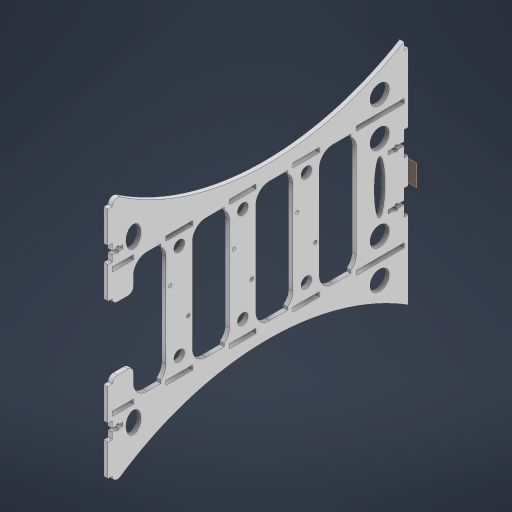
# Autodesk Inventor part: грань тела
Saved by Autodesk Inventor 2023.2 (Build 272271030, 271C)
## iProperties
Created: 2024-11-21
Part Number: грань тела
Material: Типовые
Document SubType Name: Modeling
Designer: DELL
Density: 1 g/cm^3
Appearance: По умолчанию
Author: DELL
Autodesk Inventor part; units mm, degrees
ref_plane "YZ Plane" through (0, 0, 0) normal (1, 0, 0) x (0, 1, 0)
ref_plane "XZ Plane" through (0, 0, 0) normal (0, 1, 0) x (-1, 0, 0)
ref_plane "РабПлоскость1" through (0, 0, -4) normal (0, 0, 1) x (1, 0, 0)
sketch "Эскиз10" plane through (0, 0, 0) normal (1, 0, 0) x (0, 1, 0)
  line L0 (-120, -4) -> (120, -4) construction
  line L1 (120, -4) -> (120, 276) construction
  line L2 (110.389, 276) -> (-110.389, 276)
  line L3 (-120, 276) -> (-120, -4) construction
  line L4 (-110, -4) -> (110, -4)
  arc A0 (-110, -4) -> (-114.5368, 268.208) centre (-321.9309, 128.6096) ccw
  arc A1 (114.5368, 268.208) -> (110, -4) centre (321.9309, 128.6096) ccw
  arc A2 (114.5368, 268.208) -> (110.389, 276) centre (110.389, 271) ccw
  arc A3 (-110.389, 276) -> (-114.5368, 268.208) centre (-110.389, 271) ccw
  point P0 (0, 0)
  point P1 (0, -4)
  dimension "d50" = 240
  dimension "d51" = 280
  dimension "d52" = 220
  dimension "d53" = 250
  dimension "d54" = 250
  dimension "d55" = 5
  constraints: 10 end point, 10 point on circle, 4 centre point, 4 tangent, 2 horizontal, 2 midpoint, 2 parallel, 2 point on line, 1 equal radius, 1 perpendicular
  measures "d50" distance of L3.start L1.end
  measures "d51" distance of L1.end L0.end
  measures "d52" distance of L4.start L4.end
  measures "d53" radius of A0
  measures "d54" radius of A1
  measures "d55" radius of A2
extrude "Выдавливание6" add sketch "Эскиз10" along normal mid plane 4
sketch "Эскиз12" plane through (2, 0, 0) normal (1, 0, 0) x (0, 0, -1)
  line L0 (3.3197, -100.9593) -> (0, -100.9593)
  line L1 (4, 110) -> (4, -110) projected
  line L2 (4, -110) -> (4, 110) projected
  line L3 (4, -35.9593) -> (0, -35.9593)
  line L4 (0, -35.9593) -> (0, -12.5)
  line L5 (0, -12.5) -> (4, -12.5)
  line L6 (4, 12.5) -> (0, 12.5)
  line L7 (0, 12.5) -> (0, 35.5004)
  line L8 (0, 35.5004) -> (4, 35.5004)
  line L9 (0, 100.5004) -> (4, 100.5004)
  line L10 (0, -100.9593) -> (0, -110)
  line L11 (0, -110) -> (4, -110)
  line L12 (0, 100.5004) -> (0, 110)
  line L13 (0, 110) -> (4, 110)
  line L14 (0, -100.9593) -> (0, -50.9593)
  line L15 (0, -50.9593) -> (4, -50.9593)
  line L16 (0, 100.5004) -> (0, 50.5004)
  line L17 (0, 50.5004) -> (4, 50.5004)
  point P0 (0, 0)
  point P1 (4, 12.5)
  point P2 (4, 35.5004)
  point P3 (4, -35.9593)
  point P4 (4, -12.5)
  point P5 (4, -100.9593)
  dimension "d197" = 50
  dimension "d198" = 50
  constraints: 32 end point, 11 perpendicular, 8 point on line, 3 vertical, 1 horizontal, 6 other
  measures "d197" distance of L0.end L14.end
  measures "d198" distance of L9.start L16.end
extrude "Выдавливание7" cut sketch "Эскиз12" against normal blind 4 contours L1 L9 L12 L13 | L1 L6 L7 L8 | L1 L3 L4 L5
sketch "Эскиз13" plane through (2, 0, 0) normal (1, 0, 0) x (0, 0, -1)
  line L0 (-15, -22.6546) -> (-15, -25.8046)
  line L1 (0, -25.7683) -> (0, -22.691)
  line L2 (0, -35.9593) -> (0, -12.5) projected
  line L3 (-6.1608, -27.016) -> (-8.4608, -27.016)
  line L4 (-8.4608, -21.516) -> (-6.1608, -21.516)
  line L5 (-15, -24.2296) -> (0, -24.2296) construction
  line L6 (0, -12.5) -> (0, -35.9593) projected
  line L7 (-8.4608, -27.016) -> (-8.4608, -25.8046)
  line L8 (-8.4608, -22.6546) -> (-8.4608, -21.516)
  line L9 (-15, -25.8046) -> (-8.4608, -25.8046)
  line L10 (-6.1608, -25.7683) -> (0, -25.7683)
  line L11 (-6.1608, -21.516) -> (-6.1608, -22.691)
  line L12 (-6.1608, -25.7683) -> (-6.1608, -27.016)
  line L13 (0, -22.691) -> (-6.1608, -22.691)
  line L14 (-8.4608, -22.6546) -> (-15, -22.6546)
  line L15 (0, 12.5) -> (0, 35.5004) projected
  line L16 (0, 18.7449) -> (0, 30.6124)
  line L17 (0, 22.4252) -> (0, 25.5752)
  line L18 (-15, 25.5752) -> (-15, 22.4252)
  line L19 (-8.65, 21.2502) -> (-6.35, 21.2502)
  line L20 (-6.35, 26.7502) -> (-8.65, 26.7502)
  line L21 (-15, 24.0002) -> (0, 24.0002) construction
  line L22 (-8.65, 26.7502) -> (-8.65, 25.5752)
  line L23 (-8.65, 22.4252) -> (-8.65, 21.2502)
  line L24 (-15, 22.4252) -> (-8.65, 22.4252)
  line L25 (-6.35, 22.4252) -> (0, 22.4252)
  line L26 (-6.35, 21.2502) -> (-6.35, 22.4252)
  line L27 (-6.35, 25.5752) -> (-6.35, 26.7502)
  line L28 (0, 25.5752) -> (-6.35, 25.5752)
  line L29 (-8.65, 25.5752) -> (-15, 25.5752)
  circle A0 centre (-23.1563, -40) radius 9
  line L30 (4, -35.9593) -> (4, -110) projected
  line L31 (4, 35.5004) -> (4, 100.5004) projected
  line L32 (0, 0) -> (-64.5188, 0) construction
  circle A1 centre (-23.1563, 40) radius 9
  point P0 (4, -60.9593)
  point P1 (4, 60.5004)
  dimension "d60" = 15
  dimension "d61" = 3.15
  dimension "d62" = 2.3
  dimension "d63" = 5.5
  dimension "d64" = 6.35
  dimension "d70" = 15
  dimension "d71" = 3.15
  dimension "d72" = 2.3
  dimension "d73" = 5.5
  dimension "d77" = 18
  dimension "d114" = 80
  constraints: 56 end point, 20 parallel, 10 perpendicular, 8 midpoint, 7 horizontal, 2 centre point, 2 point on line, 1 symmetric about line, 1 other
  measures "d60" distance of L1.start L0.end
  measures "d61" distance of L0.end L0.start
  measures "d62" distance of L4.start L4.end
  measures "d63" distance of L3.end L4.start
  measures "d64" distance of point (0, -24.23) L11.end
  measures "d70" distance of L18.start L17.end
  measures "d71" distance of L17.end L17.start
  measures "d72" distance of L20.end L20.start
  measures "d73" distance of L20.start L19.end
  measures "d77" diameter of A0
  measures "d114" distance of A1.centre A0.centre
extrude "Выдавливание8" cut sketch "Эскиз13" against normal blind 4
sketch "Эскиз15" plane through (-2, 0, 0) normal (-1, 0, 0) x (0, 0, 1)
  line L0 (0, 75.3813) -> (0, -75.381) construction
  line L1 (0, 57.0002) -> (0, 61.0002) construction
  line L2 (0, 61.0002) -> (276, 61.0002) construction
  line L3 (276, 61.0002) -> (276, 57.0002) construction
  line L4 (276, 57.0002) -> (0, 57.0002) construction
  line L5 (0, -61.2296) -> (0, -57.2296) construction
  line L6 (0, -57.2296) -> (276, -57.2296) construction
  line L7 (276, -57.2296) -> (276, -61.2296) construction
  line L8 (276, -61.2296) -> (0, -61.2296) construction
  circle A0 centre (23.1563, 40) radius 9 construction
  circle A1 centre (23.1563, -40) radius 9 construction
  line L9 (45.1563, 57.0002) -> (45.1563, -44.2296) construction
  line L10 (118.1563, 57.0002) -> (127.1563, 57.0002)
  line L11 (140.1563, 44.0002) -> (140.1563, -44.2296)
  line L12 (127.1563, -57.2296) -> (118.1563, -57.2296)
  line L13 (105.1563, -44.2296) -> (105.1563, 44.0002)
  line L14 (238.1563, 57.0002) -> (243, 57.0002)
  line L15 (243, -57.2296) -> (238.1563, -57.2296)
  line L16 (225.1563, -44.2296) -> (225.1563, 44.0002)
  line L17 (276, 35.0002) -> (276, 110.389)
  line L18 (178.1563, 57.0002) -> (187.1563, 57.0002)
  line L19 (200.1563, 44.0002) -> (200.1563, -44.2296)
  line L20 (187.1563, -57.2296) -> (178.1563, -57.2296)
  line L21 (165.1563, -44.2296) -> (165.1563, 44.0002)
  line L22 (58.1563, 57.0002) -> (67.1563, 57.0002)
  line L23 (80.1563, 44.0002) -> (80.1563, -44.2296)
  line L24 (67.1563, -57.2296) -> (58.1563, -57.2296)
  line L25 (45.1563, -57.2296) -> (45.1563, 44.0002)
  arc A2 (50.1563, 54.2471) -> (45.1563, 44.0002) centre (58.1563, 44.0002) ccw
  arc A3 (80.1563, 44.0002) -> (67.1563, 57.0002) centre (67.1563, 44.0002) ccw
  arc A4 (45.1563, -44.2296) -> (50.1563, -54.4766) centre (58.1563, -44.2296) ccw
  arc A5 (67.1563, -57.2296) -> (80.1563, -44.2296) centre (67.1563, -44.2296) ccw
  arc A6 (110.1563, 54.2471) -> (105.1563, 44.0002) centre (118.1563, 44.0002) ccw
  arc A7 (140.1563, 44.0002) -> (127.1563, 57.0002) centre (127.1563, 44.0002) ccw
  arc A8 (105.1563, -44.2296) -> (110.1563, -54.4766) centre (118.1563, -44.2296) ccw
  arc A9 (127.1563, -57.2296) -> (140.1563, -44.2296) centre (127.1563, -44.2296) ccw
  arc A10 (170.1563, 54.2471) -> (165.1563, 44.0002) centre (178.1563, 44.0002) ccw
  arc A11 (200.1563, 44.0002) -> (187.1563, 57.0002) centre (187.1563, 44.0002) ccw
  arc A12 (187.1563, -57.2296) -> (200.1563, -44.2296) centre (187.1563, -44.2296) ccw
  arc A13 (165.1563, -44.2296) -> (170.1563, -54.4766) centre (178.1563, -44.2296) ccw
  arc A14 (230.1563, 54.2471) -> (225.1563, 44.0002) centre (238.1563, 44.0002) ccw
  arc A15 (256, 44.0002) -> (243, 57.0002) centre (243, 44.0002) ccw
  arc A16 (243, -57.2296) -> (256, -44.2296) centre (243, -44.2296) ccw
  arc A17 (225.1563, -44.2296) -> (230.1563, -54.4766) centre (238.1563, -44.2296) ccw
  line L26 (271, -29.9962) -> (261, -29.9962)
  line L27 (261, 30.0002) -> (271, 30.0002)
  line L28 (276, -13.2762) -> (255.9998, 30.0002) construction
  line L29 (256.0015, -29.9962) -> (276, 13.2766) construction
  line L30 (276, 41.3488) -> (276, 1056.4994)
  line L31 (276, 110.389) -> (276, -110.389) projected
  arc A18 (271, 30.0002) -> (276, 35.0002) centre (271, 35.0002) ccw
  line L32 (276, -34.9962) -> (276, -49)
  arc A19 (276, -34.9962) -> (271, -29.9962) centre (271, -34.9962) ccw
  line L33 (276, 57.0002) -> (276, -57.2296)
  line L34 (256, 44.0002) -> (256, 35.0002)
  line L35 (256, -34.9962) -> (256, -44.2296)
  arc A20 (256, 35.0002) -> (261, 30.0002) centre (261, 35.0002) ccw
  arc A21 (261, -29.9962) -> (256, -34.9962) centre (261, -34.9962) ccw
  line L36 (58.1563, 57.0002) -> (50.1563, 57.0002)
  line L37 (50.1563, 57.0002) -> (50.1563, 54.2471)
  line L38 (58.1563, -57.2296) -> (50.1563, -57.2296)
  line L39 (50.1563, -57.2296) -> (50.1563, -54.4766)
  line L40 (118.1563, 57.0002) -> (110.1563, 57.0002)
  line L41 (110.1563, 57.0002) -> (110.1563, 54.2471)
  line L42 (118.1563, -57.2296) -> (110.1563, -57.2296)
  line L43 (110.1563, -57.2296) -> (110.1563, -54.4766)
  line L44 (178.1563, 57.0002) -> (170.1563, 57.0002)
  line L45 (170.1563, 57.0002) -> (170.1563, 54.2471)
  line L46 (178.1563, -57.2296) -> (170.1563, -57.2296)
  line L47 (170.1563, -57.2296) -> (170.1563, -54.4766)
  line L48 (238.1563, 57.0002) -> (230.1563, 57.0002)
  line L49 (230.1563, 54.2471) -> (230.1563, 57.0002)
  line L50 (238.1563, -57.2296) -> (230.1563, -57.2296)
  line L51 (230.1563, -57.2296) -> (230.1563, -54.4766)
  point P0 (45.1563, -57.2296)
  point P1 (105.1563, 57.0002)
  point P2 (140.1563, -57.2296)
  point P3 (225.1563, 57.0002)
  point P4 (256, -57.2296)
  point P5 (166, -0.1147)
  point P6 (165.1563, 57.0002)
  point P7 (200.1563, -57.2296)
  point P8 (80.1563, -57.2296)
  point P9 (50.1563, -52.2296)
  point P10 (269.8643, 0.0002)
  point P11 (276, 30.0002)
  point P12 (276, -29.9962)
  point P13 (256, 29.9998)
  point P14 (256, -29.9994)
  point P15 (276, -34.9998)
  point P16 (276, 35.0002)
  point P17 (45.1563, -52.2296)
  point P18 (45.1563, -55.2296)
  point P19 (45.1563, -56.2296)
  point P20 (45.1563, -42.2296)
  point P21 (45.1563, -47.2296)
  point P22 (45.1563, -44.2296)
  point P23 (230.1563, 57.0002)
  dimension "d99" = 22
  dimension "d101" = 35
  dimension "d107" = 35
  dimension "d108" = 25
  dimension "d109" = 25
  dimension "d110" = 35
  dimension "d111" = 13
  dimension "d117" = 5
  dimension "d118" = 5
  dimension "d119" = 5
  dimension "d140" = 25
  dimension "d175" = 8
  dimension "d177" = 8
  dimension "d178" = 8
  dimension "d179" = 8
  constraints: 96 end point, 41 tangent, 40 point on circle, 34 point on line, 20 centre point, 16 equal radius, 11 perpendicular, 10 parallel, 5 horizontal, 51 other
  measures "d99" distance from line of A0.centre L9
  measures "d101" distance between parallel lines of L11 L13
  measures "d107" distance between parallel lines of L21 L19
  measures "d108" distance between parallel lines of L16 L19
  measures "d109" distance between parallel lines of L21 L11
  measures "d110" distance from line of L25.start L23
  measures "d111" radius of A2
  measures "d117" radius of A18
  measures "d118" radius of A19
  measures "d119" radius of A20
  measures "d140" distance between parallel lines of L23 L13
  measures "d175" distance of L22.start L36.end
  measures "d177" distance of L24.end L38.end
  measures "d178" distance of L10.start L40.end
  measures "d179" distance of L18.start L44.end
extrude "Выдавливание10" cut sketch "Эскиз15" against normal blind 10
sketch "Эскиз18" plane through (-2, 0, 0) normal (-1, 0, 0) x (0, 0, 1)
  line L0 (276, 61.0003) -> (276, 57.0003)
  line L1 (276, -57.2293) -> (276, -61.2293)
  line L2 (225.1563, -52.2296) -> (225.1563, 52.0002) construction
  line L3 (165.1563, -52.2296) -> (165.1563, 52.0002) construction
  line L4 (105.1563, -52.2296) -> (105.1563, 52.0002) construction
  line L5 (45.1563, -52.2296) -> (45.1563, 52.0002) construction
  line L6 (45.1563, -52.2296) -> (45.1563, 52.0002) construction
  line L7 (105.1563, -52.2296) -> (105.1563, 52.0002) construction
  line L8 (225.1563, 61.0003) -> (225.1563, 57.0003)
  line L9 (225.1563, -57.2293) -> (225.1563, -61.2293)
  line L10 (165.1563, 57.0003) -> (165.1563, 61.0003)
  line L11 (165.1563, -57.2293) -> (165.1563, -61.2293)
  line L12 (105.1563, 57.0003) -> (105.1563, 61.0003)
  line L13 (105.1563, -57.2293) -> (105.1563, -61.2293)
  line L14 (45.1563, 61.0003) -> (45.1563, 57.0003)
  line L15 (45.1563, -57.2293) -> (45.1563, -61.2293)
  line L16 (80.1563, 52.0002) -> (80.1563, -52.2296) construction
  line L17 (140.1563, 44.0002) -> (140.1563, -44.2296) construction
  line L18 (200.1563, 52.0002) -> (200.1563, -52.2296) construction
  line L19 (256, 44.0002) -> (256, 35.0002) construction
  line L20 (256, -26.9962) -> (256, -44.2296) construction
  line L21 (140.1563, -44.2296) -> (140.1563, 44.0002) construction
  line L22 (200.1563, 52.0002) -> (200.1563, -52.2296) construction
  line L23 (256, 44.0002) -> (256, 35.0002) projected
  line L24 (80.1563, 61.0003) -> (80.1563, 57.0003)
  line L25 (80.1563, -57.2293) -> (80.1563, -61.2293)
  line L26 (140.1563, 61.0003) -> (140.1563, 57.0003)
  line L27 (140.1563, -57.2293) -> (140.1563, -61.2293)
  line L28 (200.1563, 61.0003) -> (200.1563, 57.0003)
  line L29 (200.1563, -57.2293) -> (200.1563, -61.2293)
  line L30 (256, -57.2293) -> (256, -61.2293)
  line L31 (256, 61.0003) -> (256, 57.0003)
  line L32 (256, 61.0003) -> (276, 61.0003)
  line L33 (276, 57.0003) -> (256, 57.0003)
  line L34 (256, -57.2293) -> (276, -57.2293)
  line L35 (276, -61.2293) -> (256, -61.2293)
  line L36 (200.1563, 61.0003) -> (225.1563, 61.0003)
  line L37 (225.1563, 57.0003) -> (200.1563, 57.0003)
  line L38 (200.1563, -57.2293) -> (225.1563, -57.2293)
  line L39 (225.1563, -61.2293) -> (200.1563, -61.2293)
  line L40 (140.1563, 61.0003) -> (165.1563, 61.0003)
  line L41 (165.1563, 57.0003) -> (140.1563, 57.0003)
  line L42 (140.1563, -57.2293) -> (165.1563, -57.2293)
  line L43 (165.1563, -61.2293) -> (140.1563, -61.2293)
  line L44 (0, 61.0003) -> (45.1563, 61.0003)
  line L45 (80.1563, 61.0003) -> (105.1563, 61.0003)
  line L46 (105.1563, 57.0003) -> (80.1563, 57.0003)
  line L47 (45.1563, 57.0003) -> (0, 57.0003)
  line L48 (0, -57.2293) -> (45.1563, -57.2293)
  line L49 (80.1563, -57.2293) -> (105.1563, -57.2293)
  line L50 (105.1563, -61.2293) -> (80.1563, -61.2293)
  line L51 (45.1563, -61.2293) -> (0, -61.2293)
  line L52 (0, 61.0003) -> (0, 57.0003)
  line L53 (0, -61.2293) -> (0, -57.2293)
  point P0 (0, 0)
  constraints: 104 end point, 2 perpendicular
extrude "Выдавливание12" cut sketch "Эскиз18" against normal blind 10
sketch "Эскиз19" plane through (-2, 0, 0) normal (-1, 0, 0) x (0, 0, 1)
  line L0 (23.1563, 40) -> (23.1563, -40) construction
  ellipse E0 centre (23.1563, 0) end of major axis (23.1563, -25) minor radius 5
  circle A0 centre (204.1563, -14.8926) radius 1.575
  circle A1 centre (221.1563, 18.2674) radius 1.575
  circle A2 centre (144.0538, -14.8926) radius 1.575
  circle A3 centre (161.0538, 18.2674) radius 1.575
  circle A4 centre (83.9062, -14.8926) radius 1.575
  circle A5 centre (100.9062, 18.2674) radius 1.575
  ellipse E1 centre (23.1563, -76.2293) end of major axis (23.1563, -85.2293) minor radius 9
  line L1 (45.1563, 44.0002) -> (45.1563, -44.2296) projected
  ellipse E2 centre (23.1563, 76.0003) end of major axis (23.1563, 67.0003) minor radius 9
  line L2 (45.1563, -61.2293) -> (0, -61.2293) projected
  line L3 (0, 61.0003) -> (45.1563, 61.0003) projected
  ellipse E3 centre (256, 76.0003) end of major axis (256, 66.0003) minor radius 7
  ellipse E4 centre (256, -76.2293) end of major axis (256, -86.2293) minor radius 7
  line L4 (256, -44.2296) -> (256, -34.9962) projected
  line L5 (256, 61.0003) -> (276, 61.0003) projected
  line L6 (276, -61.2293) -> (256, -61.2293) projected
  line L7 (276, -110.389) -> (276, -61.2293) projected
  line L8 (276, 61.0003) -> (276, 110.389) projected
  point P0 (0, 0)
  dimension "d143" = 25
  dimension "d144" = 5
  dimension "d150" = 9
  dimension "d151" = 9
  dimension "d148" = 9
  dimension "d149" = 9
  dimension "d152" = 15
  dimension "d153" = 15
  dimension "d154" = 10
  dimension "d155" = 7
  dimension "d156" = 7
  dimension "d157" = 10
  dimension "d158" = 15
  dimension "d159" = 15
  dimension "d160" = 20
  dimension "d161" = 20
  constraints: 9 centre point, 2 end point, 1 midpoint, 1 point on line, 1 tangent, 1 vertical, 6 other
  measures "d152" distance from line of L2 E1.centre
  measures "d153" distance from line of L3 point (23.156, 76)
  measures "d158" distance from line of L5 E3.centre
  measures "d159" distance from line of E4.centre L6
  measures "d160" distance from line of L7 E4.centre
  measures "d161" distance from line of L8 E3.centre
extrude "Выдавливание13" cut sketch "Эскиз19" against normal blind 10
sketch "Эскиз20" plane through (2, 0, 0) normal (1, 0, 0) x (0, 0, -1)
  circle A0 centre (-100.9062, 18.2674) radius 1.575 construction
  circle A1 centre (-83.9062, -14.8926) radius 1.575 construction
  line L0 (-100.9062, 18.2674) -> (-83.9062, 18.2674) construction
  line L1 (-83.9062, 18.2674) -> (-83.9062, -14.8926) construction
  line L2 (-83.9062, -14.8926) -> (-100.9062, -14.8926) construction
  line L3 (-100.9062, -14.8926) -> (-100.9062, 18.2674) construction
  line L4 (-92.4062, -43.3126) -> (-92.4062, 46.6874) construction
  circle A2 centre (-92.4062, -43.3126) radius 5
  circle A3 centre (-92.4062, 46.6874) radius 5
  line L5 (-100.9062, -14.8926) -> (-83.9062, 18.2674) construction
  circle A4 centre (-144.0538, -14.8926) radius 1.575 projected
  circle A5 centre (-161.0538, 18.2674) radius 1.575 projected
  line L6 (-144.0538, -14.8926) -> (-161.0538, 18.2674) construction
  line L7 (-152.5538, 46.6874) -> (-152.5538, -43.3126) construction
  circle A6 centre (-152.5538, -43.3126) radius 5
  circle A7 centre (-152.5538, 46.6874) radius 5
  circle A8 centre (-204.1563, -14.8926) radius 1.575 projected
  circle A9 centre (-221.1563, 18.2674) radius 1.575 projected
  line L8 (-204.1563, -14.8926) -> (-221.1563, 18.2674) construction
  line L9 (-212.6563, 46.6874) -> (-212.6563, -43.3126)
  circle A10 centre (-212.6563, -43.3126) radius 5
  circle A11 centre (-212.6563, 46.6874) radius 5
  point P0 (0, 0)
  point P1 (-92.4062, 1.6874)
  point P2 (-212.6563, 1.6874)
  point P3 (-152.5538, 1.6874)
  dimension "d162" = 10
  dimension "d163" = 10
  dimension "d166" = 90
  dimension "d167" = 90
  dimension "d168" = 10
  dimension "d169" = 10
  dimension "d170" = 90
  dimension "d171" = 10
  dimension "d172" = 10
  constraints: 20 end point, 6 centre point, 6 coincident, 6 midpoint, 3 vertical, 2 parallel, 1 horizontal, 1 perpendicular
  measures "d162" diameter of A2
  measures "d163" diameter of A3
  measures "d166" distance of L4.start L4.end
  measures "d167" distance of L7.start L7.end
  measures "d168" diameter of A6
  measures "d169" diameter of A7
  measures "d170" distance of L9.start L9.end
  measures "d171" diameter of A10
  measures "d172" diameter of A11
extrude "Выдавливание14" cut sketch "Эскиз20" against normal blind 4 contours A2 | A3 | A6 | A7 | A10 | A11
sketch "Эскиз21" plane through (-2, 110.389, 276) normal (0, 0, 1) x (1, 0, 0)
  line L0 (0, 0) -> (4, 0)
  line L1 (4, 0) -> (4, -30)
  line L2 (4, -30) -> (0, -30)
  line L3 (0, -30) -> (0, 0)
  line L4 (0, -220.7779) -> (4, -220.7779) projected
  line L5 (0, -220.7779) -> (4, -220.7779)
  line L6 (4, -220.7779) -> (4, -190.7779)
  line L7 (4, -190.7779) -> (0, -190.7779)
  line L8 (0, -190.7779) -> (0, -220.7779)
  line L9 (4, 0) -> (0, 0) projected
  line L10 (0, -75.3888) -> (0, -80.3888) projected
  line L11 (0, -75.3888) -> (4, -75.3888)
  line L12 (4, -75.3888) -> (4, -45.3888)
  line L13 (4, -45.3888) -> (0, -45.3888)
  line L14 (0, -45.3888) -> (0, -75.3888)
  line L15 (0, -167.6183) -> (0, -145.3852) projected
  line L16 (0, -145.3852) -> (4, -145.3852)
  line L17 (4, -145.3852) -> (4, -175.3852)
  line L18 (4, -175.3852) -> (0, -175.3852)
  line L19 (0, -175.3852) -> (0, -145.3852)
  point P0 (2, -110.389)
  point P1 (0, -2.8399)
  point P2 (2, 0)
  dimension "d180" = 4
  dimension "d181" = 30
  dimension "d182" = 4
  dimension "d183" = 30
  dimension "d184" = 4
  dimension "d185" = 30
  dimension "d186" = 4
  dimension "d187" = 30
  constraints: 32 end point, 8 parallel, 4 horizontal, 4 perpendicular, 2 midpoint
  measures "d180" distance of L1.end L2.end
  measures "d181" distance of L0.end L1.end
  measures "d182" distance of L7.end L6.end
  measures "d183" distance of L6.end L5.end
  measures "d184" distance of L13.end L12.end
  measures "d185" distance of L12.end L11.end
  measures "d186" distance of L17.end L18.end
  measures "d187" distance of L16.end L17.end
extrude "Выдавливание15" add sketch "Эскиз21" along normal blind 4
sketch "Эскиз22" plane through (-2, 0, 0) normal (-1, 0, 0) x (0, 0, 1)
  line L0 (266, 74.2696) -> (266, 71.1196)
  line L1 (276, 71.1196) -> (276, 74.2696)
  line L2 (276, 65.0002) -> (276, 80.389) projected
  line L3 (304.5543, 0) -> (244.883, 0) construction
  line L4 (272, 75.4446) -> (269.7, 75.4446)
  line L5 (269.7, 69.9446) -> (272, 69.9446)
  line L6 (272, 75.4446) -> (269.7, 69.9446) construction
  line L7 (276, 72.6946) -> (266, 72.6946) construction
  line L8 (272, 69.9446) -> (272, 71.1196)
  line L9 (272, 74.2696) -> (272, 75.4446)
  line L10 (276, 74.2696) -> (272, 74.2696)
  line L11 (269.7, 74.2696) -> (266, 74.2696)
  line L12 (269.7, 75.4446) -> (269.7, 74.2696)
  line L13 (269.7, 71.1196) -> (269.7, 69.9446)
  line L14 (266, 71.1196) -> (269.7, 71.1196)
  line L15 (272, 71.1196) -> (276, 71.1196)
  line L16 (266, -74.2696) -> (266, -71.1196)
  line L17 (276, -71.1196) -> (276, -74.2696)
  line L18 (276, -65.0002) -> (276, -80.389)
  line L19 (272, -75.4446) -> (269.7, -75.4446)
  line L20 (269.7, -69.9446) -> (272, -69.9446)
  line L21 (272, -75.4446) -> (269.7, -69.9446) construction
  line L22 (276, -72.6946) -> (266, -72.6946) construction
  line L23 (272, -69.9446) -> (272, -71.1196)
  line L24 (272, -74.2696) -> (272, -75.4446)
  line L25 (276, -74.2696) -> (272, -74.2696)
  line L26 (269.7, -74.2696) -> (266, -74.2696)
  line L27 (269.7, -75.4446) -> (269.7, -74.2696)
  line L28 (269.7, -71.1196) -> (269.7, -69.9446)
  line L29 (266, -71.1196) -> (269.7, -71.1196)
  line L30 (272, -71.1196) -> (276, -71.1196)
  point P0 (0, 0)
  point P1 (270.85, 72.6946)
  point P2 (270.85, -72.6946)
  dimension "d190" = 10
  dimension "d191" = 3.15
  dimension "d192" = 2.3
  dimension "d193" = 5.5
  constraints: 60 end point, 17 symmetric about line, 10 parallel, 4 horizontal, 4 midpoint, 4 perpendicular, 2 point on line
  measures "d190" distance of L1.start L0.end
  measures "d191" distance of L0.end L0.start
  measures "d192" distance of L4.start L4.end
  measures "d193" distance of L4.end L5.start
extrude "Выдавливание16" cut sketch "Эскиз22" against normal blind 4
